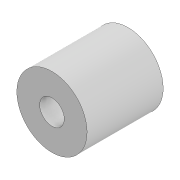
# Autodesk Inventor part: 202.001.04_Zapfen_Aktor
Saved by Autodesk Inventor 2021 (Build 250183000, 183)
## iProperties
Created: 2021-11-26
Part Number: 202.001.04_Zapfen_Aktor
Material: Generisch
Document SubType Name: Modeling
Designer: Oliver Ungerer
Density: 1 g/cm^3
Appearance: Vorgabe
Author: Oliver Ungerer
Autodesk Inventor part; units mm, degrees
ref_plane "YZ Plane" through (0, 0, 0) normal (1, 0, 0) x (0, 1, 0)
ref_plane "XZ Plane" through (0, 0, 0) normal (0, 1, 0) x (-1, 0, 0)
ref_plane "XY Plane" through (0, 0, 0) normal (0, 0, 1) x (1, 0, 0)
sketch "Skizze1" plane through (0, 0, 0) normal (1, 0, 0) x (0, 1, 0)
  line L0 (6, 0) -> (6, 13)
  line L1 (6, 13) -> (0, 13)
  line L2 (0, 13) -> (0, 0)
  line L3 (0, 0) -> (6, 0)
  dimension "d0" = 6
  dimension "d2" = 13
  constraints: 8 end point, 2 perpendicular, 1 vertical
  measures "d0" distance between parallel lines of L2 L0
  measures "d2" distance between parallel lines of L3 L1
revolve "Umdrehung1" add sketch "Skizze1" angle 360 about axis through (0, 0, 13) along (0, 0, -1)
hole "Bohrung2" at (0, 0, 0) direction (0, 0, 1) diameter 4.2 depth 13 tip angle 118
